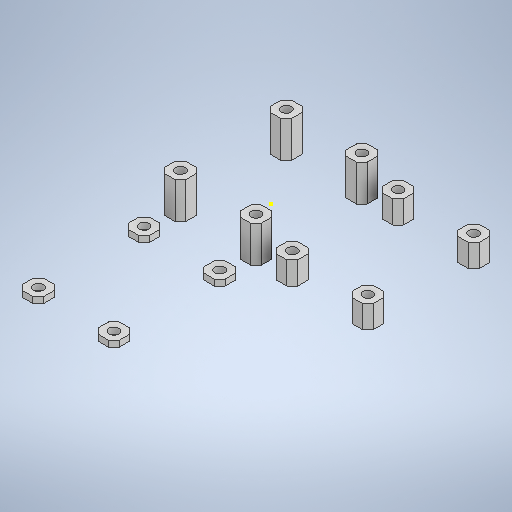
# Autodesk Inventor part: Spacer for PCB boards
Saved by Autodesk Inventor 2025 (Build 290162000, 162)
## iProperties
Created: 2024-07-10
Part Number: Spacer for PCB boards
Material: Generic
Document SubType Name: Modeling
Designer: track
Density: 1 g/cm^3
Appearance: Default
Author: track
## iProperties of the stored document Spacer for PCB boards_3DPrint.ipt
Created: 2024-07-10
Part Number: Spacer for PCB boards_3DPrint
Material: Generic
Document SubType Name: Modeling
Designer: track
Density: 1 g/cm^3
Appearance: Default
Author: track
Autodesk Inventor part; units mm, degrees
ref_plane "YZ Plane" through (0, 0, 0) normal (1, 0, 0) x (0, 1, 0)
ref_plane "XZ Plane" through (0, 0, 0) normal (0, 1, 0) x (-1, 0, 0)
ref_plane "XY Plane" through (0, 0, 0) normal (0, 0, 1) x (1, 0, 0)
sketch "Sketch1" plane through (0, 0, 0) normal (0, 1, 0) x (-1, 0, 0)
  line L0 (16, -21) -> (-16, -21)
  line L1 (-16, -21) -> (-16, 21)
  line L2 (-16, 21) -> (16, 21)
  line L3 (16, 21) -> (16, -21)
  line L4 (16, -21) -> (-16, 21) construction
  line L5 (-16, -21) -> (16, 21) construction
  line L6 (16, 21) -> (9, 21)
  line L7 (9, 21) -> (9, 14)
  line L8 (9, 14) -> (16, 14)
  line L9 (16, 14) -> (16, 21)
  line L10 (-16, 21) -> (-9, 21)
  line L11 (-9, 21) -> (-9, 14)
  line L12 (-9, 14) -> (-16, 14)
  line L13 (-16, 14) -> (-16, 21)
  line L14 (-16, -21) -> (-9, -21)
  line L15 (-9, -21) -> (-9, -14)
  line L16 (-9, -14) -> (-16, -14)
  line L17 (-16, -14) -> (-16, -21)
  line L18 (16, -21) -> (9, -21)
  line L19 (9, -21) -> (9, -14)
  line L20 (9, -14) -> (16, -14)
  line L21 (16, -14) -> (16, -21)
  circle A0 centre (12.5, 17.5) radius 1.65
  line L22 (12.5, 17.5) -> (12.5, 14) construction
  line L23 (12.5, 17.5) -> (9, 17.5) construction
  line L24 (0, 21) -> (0, -21) construction
  line L25 (-16, 0) -> (16, 0) construction
  circle A1 centre (12.5, -17.5) radius 1.65
  circle A2 centre (-12.5, 17.5) radius 1.65
  circle A3 centre (-12.5, -17.5) radius 1.65
  point P0 (0, 0)
  dimension "d0" = 42
  dimension "d1" = 32
  dimension "d9" = 7
  dimension "d10" = 7
  dimension "d11" = 7
  dimension "d12" = 7
  dimension "d13" = 7
  dimension "d14" = 7
  dimension "d15" = 7
  dimension "d16" = 3.3
  dimension "d17" = 3.5
  dimension "d18" = 3.5
  dimension "d21" = 35
  dimension "d24" = 25
  constraints: 52 end point, 10 parallel, 8 midpoint, 6 horizontal, 5 perpendicular, 4 centre point, 1 point on line, 1 vertical, 6 other
  measures "d0" distance of L2.end L0.start
  measures "d1" distance of L0.start L0.end
  measures "d9" distance between parallel lines of L19 L3
  measures "d10" distance between parallel lines of L0 L20
  measures "d11" distance of L14.end L15.end
  measures "d12" distance of L15.end L16.end
  measures "d13" distance of L11.end L12.end
  measures "d14" distance of L10.end L11.end
  measures "d15" distance of L7.end L8.end
  measures "d16" diameter of A0
  measures "d17" distance of L22.start L22.end
  measures "d18" distance of L22.start L23.end
  measures "d21" distance of L22.start A1.centre
  measures "d24" distance of L22.start A2.centre
extrude "Extrusion1" add sketch "Sketch1" along normal blind 12 contours L0 L19 L20 L3 | L0 L1 L16 L15 | L8 L7 L2 L3 | L1 L2 L11 L12
sketch "Sketch4" plane through (0, 0, 0) normal (0, 1, 0) x (-1, 0, 0)
  point P0 (0, 0)
sketch "Sketch5" plane through (0, 0, 0) normal (0, 1, 0) x (-1, 0, 0)
  line L0 (0, 0) -> (-37, 0)
  line L1 (-53, 21) -> (-21, 21)
  line L2 (-21, 21) -> (-21, -21)
  line L3 (-21, -21) -> (-53, -21)
  line L4 (-53, -21) -> (-53, 21)
  line L5 (-53, 21) -> (-21, -21) construction
  line L6 (-21, 21) -> (-53, -21) construction
  line L7 (-16, -14) -> (-16, -21) projected
  line L8 (-21, -21) -> (-28, -21)
  line L9 (-28, -21) -> (-28, -14)
  line L10 (-28, -14) -> (-21, -14)
  line L11 (-21, -14) -> (-21, -21)
  line L12 (-28, -17.5) -> (-24.5, -17.5) construction
  circle A0 centre (-24.5, -17.5) radius 1.65
  line L13 (-21, -21) -> (-21, -14)
  line L14 (-46, -21) -> (-53, -21)
  line L15 (-46, -14) -> (-46, -21)
  circle A1 centre (-49.5, -17.5) radius 1.65
  line L16 (-53, -14) -> (-46, -14)
  line L17 (-53, -21) -> (-53, -14)
  line L18 (-21, 14) -> (-28, 14)
  line L19 (-21, 21) -> (-21, 14)
  circle A2 centre (-24.5, 17.5) radius 1.65
  line L20 (-28, 21) -> (-21, 21)
  line L21 (-28, 14) -> (-28, 21)
  line L22 (-46, 14) -> (-53, 14)
  line L23 (-46, 21) -> (-46, 14)
  circle A3 centre (-49.5, 17.5) radius 1.65
  line L24 (-53, 21) -> (-46, 21)
  line L25 (-53, 14) -> (-53, 21)
  point P0 (-16, -17.5)
  point P1 (-53, -17.5)
  point P2 (-28, 17.5)
  point P3 (-53, 17.5)
  dimension "d27" = 32
  dimension "d28" = 42
  dimension "d29" = 5
  dimension "d30" = 7
  dimension "d31" = 7
  dimension "d32" = 3.3
  dimension "d33" = 3.5
  dimension "d36" = 25
  dimension "d39" = 35
  constraints: 50 end point, 5 equal length, 5 horizontal, 4 centre point, 4 midpoint, 2 perpendicular, 1 coincident, 1 vertical, 33 other
  measures "d27" distance of L2.end L3.end
  measures "d28" distance of L1.end L2.end
  measures "d29" distance from line of point (-16, -17.5) L2
  measures "d30" distance of L8.end L9.end
  measures "d31" distance of L9.end L10.end
  measures "d32" diameter of A0
  measures "d33" distance of L12.start L12.end
  measures "d36" distance of L2.end L14.start
  measures "d39" distance of L2.end L18.start
extrude "Extrusion2" add sketch "Sketch5" along normal blind 7.5 contours L1 L23 L22 L4 | L1 L2 L18 L21 | L16 L15 L3 L4 | L9 L10 L2 L3
sketch "Sketch6" plane through (0, 0, 0) normal (0, 1, 0) x (-1, 0, 0)
  line L0 (0, 0) -> (0, 47) construction
  line L1 (16, 68) -> (-16, 68)
  line L2 (-16, 68) -> (-16, 26)
  line L3 (-16, 26) -> (16, 26)
  line L4 (16, 26) -> (16, 68)
  line L5 (16, 68) -> (-16, 26) construction
  line L6 (-16, 68) -> (16, 26) construction
  line L7 (-9, 21) -> (-16, 21) projected
  line L8 (16, 26) -> (9, 26)
  line L9 (9, 26) -> (9, 33)
  line L10 (9, 33) -> (16, 33)
  line L11 (16, 33) -> (16, 26)
  line L12 (-16, 26) -> (-9, 26)
  line L13 (-16, 32.2825) -> (-16, 26)
  line L14 (12.5, 26) -> (12.5, 29.5) construction
  circle A0 centre (12.5, 29.5) radius 1.65
  line L15 (16, 33) -> (16, 26)
  line L16 (9, 26) -> (16, 26)
  circle A1 centre (-12.5, 29.5) radius 1.65
  line L17 (-16, 26) -> (-16, 33)
  line L18 (-16, 33) -> (-9, 33)
  line L19 (-9, 33) -> (-9, 26)
  line L20 (-9, 26) -> (-16, 26)
  circle A2 centre (12.5, 64.5) radius 1.65
  line L21 (9, 61) -> (9, 68)
  line L22 (9, 68) -> (16, 68)
  line L23 (16, 68) -> (16, 61)
  line L24 (16, 61) -> (9, 61)
  circle A3 centre (-12.5, 64.5) radius 1.65
  line L25 (-16, 61) -> (-16, 68)
  line L26 (-16, 68) -> (-9, 68)
  line L27 (-9, 68) -> (-9, 61)
  line L28 (-9, 61) -> (-16, 61)
  point P0 (-12.5, 26)
  point P1 (12.5, 61)
  point P2 (-12.5, 61)
  dimension "d44" = 32
  dimension "d45" = 42
  dimension "d47" = 5
  dimension "d48" = 7
  dimension "d49" = 7
  dimension "d50" = 3.3
  dimension "d51" = 3.5
  dimension "d54" = 25
  dimension "d57" = 35
  constraints: 56 end point, 5 equal length, 4 centre point, 4 horizontal, 3 midpoint, 3 perpendicular, 3 vertical, 1 coincident, 33 other
  measures "d44" distance of L2.end L3.end
  measures "d45" distance of L1.end L2.end
  measures "d47" distance between parallel lines of L7 L3
  measures "d48" distance of L8.end L9.end
  measures "d49" distance of L9.end L10.end
  measures "d50" diameter of A0
  measures "d51" distance of L14.start L14.end
  measures "d54" distance of A0.centre A1.centre
  measures "d57" distance of A0.centre A2.centre
extrude "Extrusion3" add sketch "Sketch6" along normal blind 2 contours L4 L24 L21 L1 | L27 L28 L2 L1 | L4 L3 L9 L10 | L18 L19 L3 L2
chamfer "Chamfer1" distance 1.75 angle 45 48 edges at (16, 6, 21) (9, 6, 21) (16, 6, 14) (9, 6, 14) (16, 1, 26) (16, 1, 33) (9, 1, 33) (9, 1, 26) (21, 3.75, 21) (21, 3.75, 14) (28, 3.75, 21) (28, 3.75, 14) (53, 3.75, 14) (53, 3.75, 21) (46, 3.75, 21) (46, 3.75, 14) (9, 1, 68) (9, 1, 61) (16, 1, 61) (16, 1, 68) (-9, 1, 68) (-16, 1, 68) (-16, 1, 61) (-9, 1, 61) (-9, 1, 33) (-9, 1, 26) (-16, 1, 26) (-16, 1, 33) (-9, 6, 21) (-9, 6, 14) (-16, 6, 21) (-16, 6, 14) (-9, 6, -14) (-9, 6, -21) (-16, 6, -14) (-16, 6, -21) (16, 6, -14) (16, 6, -21) (9, 6, -14) (9, 6, -21) (28, 3.75, -14) (28, 3.75, -21) (21, 3.75, -14) (21, 3.75, -21) (53, 3.75, -14) (53, 3.75, -21) (46, 3.75, -21) (46, 3.75, -14)
body "Solid1"
